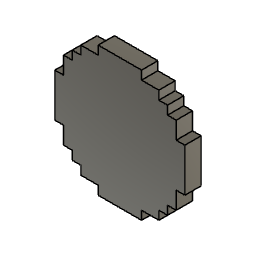
Normal Disc (Autodesk Fusion 360 design; units mm, degrees)
Autodesk Fusion 360 part; units mm, degrees
sketch "Sketch1" plane through (0, 0, 0) normal (0, 1, 0) x (1, 0, 0)
  line L0 (0, 0) -> (-8, 0)
  line L1 (0, 0) -> (0, -8)
  line L2 (0, 0) -> (8, 0)
  line L3 (8, 0) -> (8, -8)
  line L4 (8, -8) -> (0, -8)
  line L5 (0, -8) -> (0, 0)
  line L6 (8, -8) -> (8, 0)
  line L7 (8, 0) -> (16, 0)
  line L8 (16, 0) -> (16, -8)
  line L9 (16, -8) -> (8, -8)
  line L10 (16, -8) -> (16, 0)
  line L11 (16, 0) -> (24, 0)
  line L12 (24, 0) -> (24, -8)
  line L13 (24, -8) -> (16, -8)
  line L14 (24, -8) -> (24, 0)
  line L15 (24, 0) -> (32, 0)
  line L16 (32, 0) -> (32, -8)
  line L17 (32, -8) -> (24, -8)
  line L18 (32, -8) -> (32, 0)
  line L19 (32, 0) -> (40, 0)
  line L20 (40, 0) -> (40, -8)
  line L21 (40, -8) -> (32, -8)
  line L22 (40, -8) -> (40, 0)
  line L23 (40, 0) -> (48, 0)
  line L24 (48, 0) -> (48, -8)
  line L25 (48, -8) -> (40, -8)
  line L26 (48, -8) -> (48, 0)
  line L27 (48, 0) -> (56, 0)
  line L28 (56, 0) -> (56, -8)
  line L29 (56, -8) -> (48, -8)
  line L30 (56, -8) -> (56, 0)
  line L31 (56, 0) -> (64, 0)
  line L32 (64, 0) -> (64, -8)
  line L33 (64, -8) -> (56, -8)
  line L34 (64, -8) -> (64, 0)
  line L35 (64, 0) -> (72, 0)
  line L36 (72, 0) -> (72, -8)
  line L37 (72, -8) -> (64, -8)
  line L38 (72, -8) -> (72, 0)
  line L39 (72, 0) -> (80, 0)
  line L40 (80, 0) -> (80, -8)
  line L41 (80, -8) -> (72, -8)
  line L42 (80, -8) -> (80, 0)
  line L43 (80, 0) -> (88, 0)
  line L44 (88, 0) -> (88, -8)
  line L45 (88, -8) -> (80, -8)
  line L46 (88, -8) -> (88, 0)
  line L47 (88, 0) -> (96, 0)
  line L48 (96, 0) -> (96, -8)
  line L49 (96, -8) -> (88, -8)
  line L50 (96, -8) -> (96, 0)
  line L51 (96, 0) -> (104, 0)
  line L52 (104, 0) -> (104, -8)
  line L53 (104, -8) -> (96, -8)
  line L54 (104, -8) -> (104, 0)
  line L55 (104, 0) -> (112, 0)
  line L56 (112, 0) -> (112, -8)
  line L57 (112, -8) -> (104, -8)
  line L58 (112, -8) -> (112, 0)
  line L59 (112, 0) -> (120, 0)
  line L60 (120, 0) -> (120, -8)
  line L61 (120, -8) -> (112, -8)
  line L62 (32, -8) -> (32, -16)
  line L63 (72, -8) -> (72, -16)
  line L64 (8, -16) -> (8, -8)
  line L65 (32, -16) -> (32, -8)
  line L66 (64, -8) -> (64, -16)
  line L67 (80, -8) -> (80, -16)
  line L68 (32, -8) -> (40, -8)
  line L69 (8, -8) -> (16, -8)
  line L70 (56, -16) -> (56, -8)
  line L71 (80, -16) -> (80, -8)
  line L72 (64, -8) -> (72, -8)
  line L73 (96, -8) -> (96, -16)
  line L74 (48, -8) -> (56, -8)
  line L75 (88, -16) -> (88, -8)
  line L76 (48, -8) -> (48, -16)
  line L77 (0, -16) -> (0, -8)
  line L78 (104, -8) -> (104, -16)
  line L79 (88, -8) -> (88, -16)
  line L80 (24, -8) -> (32, -8)
  line L81 (16, -8) -> (24, -8)
  line L82 (8, -8) -> (8, -16)
  line L83 (0, -8) -> (8, -8)
  line L84 (88, -8) -> (96, -8)
  line L85 (24, -16) -> (24, -8)
  line L86 (48, -16) -> (48, -8)
  line L87 (56, -8) -> (64, -8)
  line L88 (16, -8) -> (16, -16)
  line L89 (24, -8) -> (24, -16)
  line L90 (80, -8) -> (88, -8)
  line L91 (96, -8) -> (104, -8)
  line L92 (40, -8) -> (40, -16)
  line L93 (72, -16) -> (72, -8)
  line L94 (104, -16) -> (104, -8)
  line L95 (64, -16) -> (64, -8)
  line L96 (40, -16) -> (40, -8)
  line L97 (104, -8) -> (112, -8)
  line L98 (96, -16) -> (96, -8)
  line L99 (72, -8) -> (80, -8)
  line L100 (56, -8) -> (56, -16)
  line L101 (16, -16) -> (16, -8)
  line L102 (0, -8) -> (0, -16)
  line L103 (40, -8) -> (48, -8)
  line L104 (104, -16) -> (96, -16)
  line L105 (112, -16) -> (104, -16)
  line L106 (96, -16) -> (88, -16)
  line L107 (64, -16) -> (56, -16)
  line L108 (120, -16) -> (112, -16)
  line L109 (24, -16) -> (16, -16)
  line L110 (88, -16) -> (80, -16)
  line L111 (56, -16) -> (48, -16)
  line L112 (72, -16) -> (64, -16)
  line L113 (80, -16) -> (72, -16)
  line L114 (40, -16) -> (32, -16)
  line L115 (32, -16) -> (24, -16)
  line L116 (8, -16) -> (0, -16)
  line L117 (48, -16) -> (40, -16)
  line L118 (16, -16) -> (8, -16)
  line L119 (120, -8) -> (120, -16)
  line L120 (112, -8) -> (120, -8)
  line L121 (112, -16) -> (112, -8)
  line L122 (32, -16) -> (32, -24)
  line L123 (72, -16) -> (72, -24)
  line L124 (8, -24) -> (8, -16)
  line L125 (32, -24) -> (32, -16)
  line L126 (64, -16) -> (64, -24)
  line L127 (80, -16) -> (80, -24)
  line L128 (32, -16) -> (40, -16)
  line L129 (8, -16) -> (16, -16)
  line L130 (56, -24) -> (56, -16)
  line L131 (80, -24) -> (80, -16)
  line L132 (64, -16) -> (72, -16)
  line L133 (96, -16) -> (96, -24)
  line L134 (48, -16) -> (56, -16)
  line L135 (88, -24) -> (88, -16)
  line L136 (48, -16) -> (48, -24)
  line L137 (0, -24) -> (0, -16)
  line L138 (104, -16) -> (104, -24)
  line L139 (88, -16) -> (88, -24)
  line L140 (24, -16) -> (32, -16)
  line L141 (16, -16) -> (24, -16)
  line L142 (8, -16) -> (8, -24)
  line L143 (0, -16) -> (8, -16)
  line L144 (88, -16) -> (96, -16)
  line L145 (24, -24) -> (24, -16)
  line L146 (48, -24) -> (48, -16)
  line L147 (56, -16) -> (64, -16)
  line L148 (16, -16) -> (16, -24)
  line L149 (24, -16) -> (24, -24)
  line L150 (80, -16) -> (88, -16)
  line L151 (96, -16) -> (104, -16)
  line L152 (40, -16) -> (40, -24)
  line L153 (72, -24) -> (72, -16)
  line L154 (104, -24) -> (104, -16)
  line L155 (64, -24) -> (64, -16)
  line L156 (40, -24) -> (40, -16)
  line L157 (104, -16) -> (112, -16)
  line L158 (96, -24) -> (96, -16)
  line L159 (72, -16) -> (80, -16)
  line L160 (56, -16) -> (56, -24)
  line L161 (16, -24) -> (16, -16)
  line L162 (0, -16) -> (0, -24)
  line L163 (40, -16) -> (48, -16)
  line L164 (104, -24) -> (96, -24)
  line L165 (112, -24) -> (104, -24)
  line L166 (96, -24) -> (88, -24)
  line L167 (64, -24) -> (56, -24)
  line L168 (120, -24) -> (112, -24)
  line L169 (24, -24) -> (16, -24)
  line L170 (88, -24) -> (80, -24)
  line L171 (56, -24) -> (48, -24)
  line L172 (72, -24) -> (64, -24)
  line L173 (80, -24) -> (72, -24)
  line L174 (40, -24) -> (32, -24)
  line L175 (32, -24) -> (24, -24)
  line L176 (8, -24) -> (0, -24)
  line L177 (48, -24) -> (40, -24)
  line L178 (16, -24) -> (8, -24)
  line L179 (120, -16) -> (120, -24)
  line L180 (112, -16) -> (120, -16)
  line L181 (112, -24) -> (112, -16)
  line L182 (32, -24) -> (32, -32)
  line L183 (72, -24) -> (72, -32)
  line L184 (8, -32) -> (8, -24)
  line L185 (32, -32) -> (32, -24)
  line L186 (64, -24) -> (64, -32)
  line L187 (80, -24) -> (80, -32)
  line L188 (32, -24) -> (40, -24)
  line L189 (8, -24) -> (16, -24)
  line L190 (56, -32) -> (56, -24)
  line L191 (80, -32) -> (80, -24)
  line L192 (64, -24) -> (72, -24)
  line L193 (96, -24) -> (96, -32)
  line L194 (48, -24) -> (56, -24)
  line L195 (88, -32) -> (88, -24)
  line L196 (48, -24) -> (48, -32)
  line L197 (0, -32) -> (0, -24)
  line L198 (104, -24) -> (104, -32)
  line L199 (88, -24) -> (88, -32)
  line L200 (24, -24) -> (32, -24)
  line L201 (16, -24) -> (24, -24)
  line L202 (8, -24) -> (8, -32)
  line L203 (0, -24) -> (8, -24)
  line L204 (88, -24) -> (96, -24)
  line L205 (24, -32) -> (24, -24)
  line L206 (48, -32) -> (48, -24)
  line L207 (56, -24) -> (64, -24)
  line L208 (16, -24) -> (16, -32)
  line L209 (24, -24) -> (24, -32)
  line L210 (80, -24) -> (88, -24)
  line L211 (96, -24) -> (104, -24)
  line L212 (40, -24) -> (40, -32)
  line L213 (72, -32) -> (72, -24)
  line L214 (104, -32) -> (104, -24)
  line L215 (64, -32) -> (64, -24)
  line L216 (40, -32) -> (40, -24)
  line L217 (104, -24) -> (112, -24)
  line L218 (96, -32) -> (96, -24)
  line L219 (72, -24) -> (80, -24)
  line L220 (56, -24) -> (56, -32)
  line L221 (16, -32) -> (16, -24)
  line L222 (0, -24) -> (0, -32)
  line L223 (40, -24) -> (48, -24)
  line L224 (104, -32) -> (96, -32)
  line L225 (112, -32) -> (104, -32)
  line L226 (96, -32) -> (88, -32)
  line L227 (64, -32) -> (56, -32)
  line L228 (120, -32) -> (112, -32)
  line L229 (24, -32) -> (16, -32)
  line L230 (88, -32) -> (80, -32)
  line L231 (56, -32) -> (48, -32)
  line L232 (72, -32) -> (64, -32)
  line L233 (80, -32) -> (72, -32)
  line L234 (40, -32) -> (32, -32)
  line L235 (32, -32) -> (24, -32)
  line L236 (8, -32) -> (0, -32)
  line L237 (48, -32) -> (40, -32)
  line L238 (16, -32) -> (8, -32)
  line L239 (120, -24) -> (120, -32)
  line L240 (112, -24) -> (120, -24)
  line L241 (112, -32) -> (112, -24)
  line L242 (32, -32) -> (32, -40)
  line L243 (72, -32) -> (72, -40)
  line L244 (8, -40) -> (8, -32)
  line L245 (32, -40) -> (32, -32)
  line L246 (64, -32) -> (64, -40)
  line L247 (80, -32) -> (80, -40)
  line L248 (32, -32) -> (40, -32)
  line L249 (8, -32) -> (16, -32)
  line L250 (56, -40) -> (56, -32)
  line L251 (80, -40) -> (80, -32)
  line L252 (64, -32) -> (72, -32)
  line L253 (96, -32) -> (96, -40)
  line L254 (48, -32) -> (56, -32)
  line L255 (88, -40) -> (88, -32)
  line L256 (48, -32) -> (48, -40)
  line L257 (0, -40) -> (0, -32)
  line L258 (104, -32) -> (104, -40)
  line L259 (88, -32) -> (88, -40)
  line L260 (24, -32) -> (32, -32)
  line L261 (16, -32) -> (24, -32)
  line L262 (8, -32) -> (8, -40)
  line L263 (0, -32) -> (8, -32)
  line L264 (88, -32) -> (96, -32)
  line L265 (24, -40) -> (24, -32)
  line L266 (48, -40) -> (48, -32)
  line L267 (56, -32) -> (64, -32)
  line L268 (16, -32) -> (16, -40)
  line L269 (24, -32) -> (24, -40)
  line L270 (80, -32) -> (88, -32)
  line L271 (96, -32) -> (104, -32)
  line L272 (40, -32) -> (40, -40)
  line L273 (72, -40) -> (72, -32)
  line L274 (104, -40) -> (104, -32)
  line L275 (64, -40) -> (64, -32)
  line L276 (40, -40) -> (40, -32)
  line L277 (104, -32) -> (112, -32)
  line L278 (96, -40) -> (96, -32)
  line L279 (72, -32) -> (80, -32)
  line L280 (56, -32) -> (56, -40)
  line L281 (16, -40) -> (16, -32)
  line L282 (0, -32) -> (0, -40)
  line L283 (40, -32) -> (48, -32)
  line L284 (104, -40) -> (96, -40)
  line L285 (112, -40) -> (104, -40)
  line L286 (96, -40) -> (88, -40)
  line L287 (64, -40) -> (56, -40)
  line L288 (120, -40) -> (112, -40)
  line L289 (24, -40) -> (16, -40)
  line L290 (88, -40) -> (80, -40)
  line L291 (56, -40) -> (48, -40)
  line L292 (72, -40) -> (64, -40)
  line L293 (80, -40) -> (72, -40)
  line L294 (40, -40) -> (32, -40)
  line L295 (32, -40) -> (24, -40)
  line L296 (8, -40) -> (0, -40)
  line L297 (48, -40) -> (40, -40)
  line L298 (16, -40) -> (8, -40)
  line L299 (120, -32) -> (120, -40)
  line L300 (112, -32) -> (120, -32)
  line L301 (112, -40) -> (112, -32)
  line L302 (32, -40) -> (32, -48)
  line L303 (72, -40) -> (72, -48)
  line L304 (8, -48) -> (8, -40)
  line L305 (32, -48) -> (32, -40)
  line L306 (64, -40) -> (64, -48)
  line L307 (80, -40) -> (80, -48)
  line L308 (32, -40) -> (40, -40)
  line L309 (8, -40) -> (16, -40)
  line L310 (56, -48) -> (56, -40)
  line L311 (80, -48) -> (80, -40)
  line L312 (64, -40) -> (72, -40)
  line L313 (96, -40) -> (96, -48)
  line L314 (48, -40) -> (56, -40)
  line L315 (88, -48) -> (88, -40)
  line L316 (48, -40) -> (48, -48)
  line L317 (0, -48) -> (0, -40)
  line L318 (104, -40) -> (104, -48)
  line L319 (88, -40) -> (88, -48)
  line L320 (24, -40) -> (32, -40)
  line L321 (16, -40) -> (24, -40)
  line L322 (8, -40) -> (8, -48)
  line L323 (0, -40) -> (8, -40)
  line L324 (88, -40) -> (96, -40)
  line L325 (24, -48) -> (24, -40)
  line L326 (48, -48) -> (48, -40)
  line L327 (56, -40) -> (64, -40)
  line L328 (16, -40) -> (16, -48)
  line L329 (24, -40) -> (24, -48)
  line L330 (80, -40) -> (88, -40)
  line L331 (96, -40) -> (104, -40)
  line L332 (40, -40) -> (40, -48)
  line L333 (72, -48) -> (72, -40)
  line L334 (104, -48) -> (104, -40)
  line L335 (64, -48) -> (64, -40)
  line L336 (40, -48) -> (40, -40)
  line L337 (104, -40) -> (112, -40)
  line L338 (96, -48) -> (96, -40)
  line L339 (72, -40) -> (80, -40)
  line L340 (56, -40) -> (56, -48)
  line L341 (16, -48) -> (16, -40)
  line L342 (0, -40) -> (0, -48)
  line L343 (40, -40) -> (48, -40)
  line L344 (104, -48) -> (96, -48)
  line L345 (112, -48) -> (104, -48)
  line L346 (96, -48) -> (88, -48)
  line L347 (64, -48) -> (56, -48)
  line L348 (120, -48) -> (112, -48)
  line L349 (24, -48) -> (16, -48)
  line L350 (88, -48) -> (80, -48)
  line L351 (56, -48) -> (48, -48)
  line L352 (72, -48) -> (64, -48)
  line L353 (80, -48) -> (72, -48)
  line L354 (40, -48) -> (32, -48)
  line L355 (32, -48) -> (24, -48)
  line L356 (8, -48) -> (0, -48)
  line L357 (48, -48) -> (40, -48)
  line L358 (16, -48) -> (8, -48)
  line L359 (120, -40) -> (120, -48)
  line L360 (112, -40) -> (120, -40)
  line L361 (112, -48) -> (112, -40)
  line L362 (32, -48) -> (32, -56)
  line L363 (72, -48) -> (72, -56)
  line L364 (8, -56) -> (8, -48)
  line L365 (32, -56) -> (32, -48)
  line L366 (64, -48) -> (64, -56)
  line L367 (80, -48) -> (80, -56)
  line L368 (32, -48) -> (40, -48)
  line L369 (8, -48) -> (16, -48)
  line L370 (56, -56) -> (56, -48)
  line L371 (80, -56) -> (80, -48)
  line L372 (64, -48) -> (72, -48)
  line L373 (96, -48) -> (96, -56)
  line L374 (48, -48) -> (56, -48)
  line L375 (88, -56) -> (88, -48)
  line L376 (48, -48) -> (48, -56)
  line L377 (0, -56) -> (0, -48)
  line L378 (104, -48) -> (104, -56)
  line L379 (88, -48) -> (88, -56)
  line L380 (24, -48) -> (32, -48)
  line L381 (16, -48) -> (24, -48)
  line L382 (8, -48) -> (8, -56)
  line L383 (0, -48) -> (8, -48)
  line L384 (88, -48) -> (96, -48)
  line L385 (24, -56) -> (24, -48)
  line L386 (48, -56) -> (48, -48)
  line L387 (56, -48) -> (64, -48)
  line L388 (16, -48) -> (16, -56)
  line L389 (24, -48) -> (24, -56)
  line L390 (80, -48) -> (88, -48)
  line L391 (96, -48) -> (104, -48)
  line L392 (40, -48) -> (40, -56)
  line L393 (72, -56) -> (72, -48)
  line L394 (104, -56) -> (104, -48)
  line L395 (64, -56) -> (64, -48)
  line L396 (40, -56) -> (40, -48)
  line L397 (104, -48) -> (112, -48)
  line L398 (96, -56) -> (96, -48)
  line L399 (72, -48) -> (80, -48)
  line L400 (56, -48) -> (56, -56)
  line L401 (16, -56) -> (16, -48)
  line L402 (0, -48) -> (0, -56)
  line L403 (40, -48) -> (48, -48)
  line L404 (104, -56) -> (96, -56)
  line L405 (112, -56) -> (104, -56)
  line L406 (96, -56) -> (88, -56)
  line L407 (64, -56) -> (56, -56)
  line L408 (120, -56) -> (112, -56)
  line L409 (24, -56) -> (16, -56)
  line L410 (88, -56) -> (80, -56)
  line L411 (56, -56) -> (48, -56)
  line L412 (72, -56) -> (64, -56)
  line L413 (80, -56) -> (72, -56)
  line L414 (40, -56) -> (32, -56)
  line L415 (32, -56) -> (24, -56)
  line L416 (8, -56) -> (0, -56)
  line L417 (48, -56) -> (40, -56)
  line L418 (16, -56) -> (8, -56)
  line L419 (120, -48) -> (120, -56)
  line L420 (112, -48) -> (120, -48)
  line L421 (112, -56) -> (112, -48)
  line L422 (32, -56) -> (32, -64)
  line L423 (72, -56) -> (72, -64)
  line L424 (8, -64) -> (8, -56)
  line L425 (32, -64) -> (32, -56)
  line L426 (64, -56) -> (64, -64)
  line L427 (80, -56) -> (80, -64)
  line L428 (32, -56) -> (40, -56)
  line L429 (8, -56) -> (16, -56)
  line L430 (56, -64) -> (56, -56)
  line L431 (80, -64) -> (80, -56)
  line L432 (64, -56) -> (72, -56)
  line L433 (96, -56) -> (96, -64)
  line L434 (48, -56) -> (56, -56)
  line L435 (88, -64) -> (88, -56)
  line L436 (48, -56) -> (48, -64)
  line L437 (0, -64) -> (0, -56)
  line L438 (104, -56) -> (104, -64)
  line L439 (88, -56) -> (88, -64)
  line L440 (24, -56) -> (32, -56)
  line L441 (16, -56) -> (24, -56)
  line L442 (8, -56) -> (8, -64)
  line L443 (0, -56) -> (8, -56)
  line L444 (88, -56) -> (96, -56)
  line L445 (24, -64) -> (24, -56)
  line L446 (48, -64) -> (48, -56)
  line L447 (56, -56) -> (64, -56)
  line L448 (16, -56) -> (16, -64)
  line L449 (24, -56) -> (24, -64)
  line L450 (80, -56) -> (88, -56)
  line L451 (96, -56) -> (104, -56)
  line L452 (40, -56) -> (40, -64)
  line L453 (72, -64) -> (72, -56)
  line L454 (104, -64) -> (104, -56)
  line L455 (64, -64) -> (64, -56)
  line L456 (40, -64) -> (40, -56)
  line L457 (104, -56) -> (112, -56)
  line L458 (96, -64) -> (96, -56)
  line L459 (72, -56) -> (80, -56)
  line L460 (56, -56) -> (56, -64)
  line L461 (16, -64) -> (16, -56)
  line L462 (0, -56) -> (0, -64)
  line L463 (40, -56) -> (48, -56)
  line L464 (104, -64) -> (96, -64)
  line L465 (112, -64) -> (104, -64)
  line L466 (96, -64) -> (88, -64)
  line L467 (64, -64) -> (56, -64)
  line L468 (120, -64) -> (112, -64)
  line L469 (24, -64) -> (16, -64)
  line L470 (88, -64) -> (80, -64)
  line L471 (56, -64) -> (48, -64)
  line L472 (72, -64) -> (64, -64)
  line L473 (80, -64) -> (72, -64)
  line L474 (40, -64) -> (32, -64)
  line L475 (32, -64) -> (24, -64)
  line L476 (8, -64) -> (0, -64)
  line L477 (48, -64) -> (40, -64)
  line L478 (16, -64) -> (8, -64)
  line L479 (120, -56) -> (120, -64)
  line L480 (112, -56) -> (120, -56)
  line L481 (112, -64) -> (112, -56)
  line L482 (32, -64) -> (32, -72)
  line L483 (72, -64) -> (72, -72)
  line L484 (8, -72) -> (8, -64)
  line L485 (32, -72) -> (32, -64)
  line L486 (64, -64) -> (64, -72)
  line L487 (80, -64) -> (80, -72)
  line L488 (32, -64) -> (40, -64)
  line L489 (8, -64) -> (16, -64)
  line L490 (56, -72) -> (56, -64)
  line L491 (80, -72) -> (80, -64)
  line L492 (64, -64) -> (72, -64)
  line L493 (96, -64) -> (96, -72)
  line L494 (48, -64) -> (56, -64)
  line L495 (88, -72) -> (88, -64)
  line L496 (48, -64) -> (48, -72)
  line L497 (0, -72) -> (0, -64)
  line L498 (104, -64) -> (104, -72)
  line L499 (88, -64) -> (88, -72)
  line L500 (24, -64) -> (32, -64)
  line L501 (16, -64) -> (24, -64)
  line L502 (8, -64) -> (8, -72)
  line L503 (0, -64) -> (8, -64)
  line L504 (88, -64) -> (96, -64)
  line L505 (24, -72) -> (24, -64)
  line L506 (48, -72) -> (48, -64)
  line L507 (56, -64) -> (64, -64)
  line L508 (16, -64) -> (16, -72)
  line L509 (24, -64) -> (24, -72)
  line L510 (80, -64) -> (88, -64)
  line L511 (96, -64) -> (104, -64)
  line L512 (40, -64) -> (40, -72)
  line L513 (72, -72) -> (72, -64)
  line L514 (104, -72) -> (104, -64)
  line L515 (64, -72) -> (64, -64)
  line L516 (40, -72) -> (40, -64)
  line L517 (104, -64) -> (112, -64)
  line L518 (96, -72) -> (96, -64)
  line L519 (72, -64) -> (80, -64)
  line L520 (56, -64) -> (56, -72)
  line L521 (16, -72) -> (16, -64)
  line L522 (0, -64) -> (0, -72)
  line L523 (40, -64) -> (48, -64)
  line L524 (104, -72) -> (96, -72)
  line L525 (112, -72) -> (104, -72)
  line L526 (96, -72) -> (88, -72)
  line L527 (64, -72) -> (56, -72)
  line L528 (120, -72) -> (112, -72)
  line L529 (24, -72) -> (16, -72)
  line L530 (88, -72) -> (80, -72)
  line L531 (56, -72) -> (48, -72)
  line L532 (72, -72) -> (64, -72)
  line L533 (80, -72) -> (72, -72)
  line L534 (40, -72) -> (32, -72)
  line L535 (32, -72) -> (24, -72)
  line L536 (8, -72) -> (0, -72)
  line L537 (48, -72) -> (40, -72)
  line L538 (16, -72) -> (8, -72)
  line L539 (120, -64) -> (120, -72)
  line L540 (112, -64) -> (120, -64)
  line L541 (112, -72) -> (112, -64)
  line L542 (32, -72) -> (32, -80)
  line L543 (72, -72) -> (72, -80)
  line L544 (8, -80) -> (8, -72)
  line L545 (32, -80) -> (32, -72)
  line L546 (64, -72) -> (64, -80)
  line L547 (80, -72) -> (80, -80)
  line L548 (32, -72) -> (40, -72)
  line L549 (8, -72) -> (16, -72)
  line L550 (56, -80) -> (56, -72)
  line L551 (80, -80) -> (80, -72)
  line L552 (64, -72) -> (72, -72)
  line L553 (96, -72) -> (96, -80)
  line L554 (48, -72) -> (56, -72)
  line L555 (88, -80) -> (88, -72)
  line L556 (48, -72) -> (48, -80)
  line L557 (0, -80) -> (0, -72)
  line L558 (104, -72) -> (104, -80)
  line L559 (88, -72) -> (88, -80)
  line L560 (24, -72) -> (32, -72)
  line L561 (16, -72) -> (24, -72)
  line L562 (8, -72) -> (8, -80)
  line L563 (0, -72) -> (8, -72)
  line L564 (88, -72) -> (96, -72)
  line L565 (24, -80) -> (24, -72)
  line L566 (48, -80) -> (48, -72)
  line L567 (56, -72) -> (64, -72)
  line L568 (16, -72) -> (16, -80)
  line L569 (24, -72) -> (24, -80)
  line L570 (80, -72) -> (88, -72)
  line L571 (96, -72) -> (104, -72)
  line L572 (40, -72) -> (40, -80)
  line L573 (72, -80) -> (72, -72)
  line L574 (104, -80) -> (104, -72)
  line L575 (64, -80) -> (64, -72)
  line L576 (40, -80) -> (40, -72)
  line L577 (104, -72) -> (112, -72)
  line L578 (96, -80) -> (96, -72)
  line L579 (72, -72) -> (80, -72)
  line L580 (56, -72) -> (56, -80)
  line L581 (16, -80) -> (16, -72)
  line L582 (0, -72) -> (0, -80)
  line L583 (40, -72) -> (48, -72)
  line L584 (104, -80) -> (96, -80)
  line L585 (112, -80) -> (104, -80)
  line L586 (96, -80) -> (88, -80)
  line L587 (64, -80) -> (56, -80)
  line L588 (120, -80) -> (112, -80)
  line L589 (24, -80) -> (16, -80)
  line L590 (88, -80) -> (80, -80)
  line L591 (56, -80) -> (48, -80)
  line L592 (72, -80) -> (64, -80)
  line L593 (80, -80) -> (72, -80)
  line L594 (40, -80) -> (32, -80)
  line L595 (32, -80) -> (24, -80)
  line L596 (8, -80) -> (0, -80)
  line L597 (48, -80) -> (40, -80)
  line L598 (16, -80) -> (8, -80)
  line L599 (120, -72) -> (120, -80)
  line L600 (112, -72) -> (120, -72)
  line L601 (112, -80) -> (112, -72)
  line L602 (32, -80) -> (32, -88)
  line L603 (72, -80) -> (72, -88)
  line L604 (8, -88) -> (8, -80)
  line L605 (32, -88) -> (32, -80)
  line L606 (64, -80) -> (64, -88)
  line L607 (80, -80) -> (80, -88)
  line L608 (32, -80) -> (40, -80)
  line L609 (8, -80) -> (16, -80)
  line L610 (56, -88) -> (56, -80)
  line L611 (80, -88) -> (80, -80)
  line L612 (64, -80) -> (72, -80)
  line L613 (96, -80) -> (96, -88)
  line L614 (48, -80) -> (56, -80)
  line L615 (88, -88) -> (88, -80)
  line L616 (48, -80) -> (48, -88)
  line L617 (0, -88) -> (0, -80)
  line L618 (104, -80) -> (104, -88)
  line L619 (88, -80) -> (88, -88)
  line L620 (24, -80) -> (32, -80)
  line L621 (16, -80) -> (24, -80)
  line L622 (8, -80) -> (8, -88)
  line L623 (0, -80) -> (8, -80)
  line L624 (88, -80) -> (96, -80)
  line L625 (24, -88) -> (24, -80)
  line L626 (48, -88) -> (48, -80)
  line L627 (56, -80) -> (64, -80)
  line L628 (16, -80) -> (16, -88)
  line L629 (24, -80) -> (24, -88)
  line L630 (80, -80) -> (88, -80)
  line L631 (96, -80) -> (104, -80)
  line L632 (40, -80) -> (40, -88)
  line L633 (72, -88) -> (72, -80)
  line L634 (104, -88) -> (104, -80)
  line L635 (64, -88) -> (64, -80)
  line L636 (40, -88) -> (40, -80)
  line L637 (104, -80) -> (112, -80)
  line L638 (96, -88) -> (96, -80)
  line L639 (72, -80) -> (80, -80)
  line L640 (56, -80) -> (56, -88)
  line L641 (16, -88) -> (16, -80)
  line L642 (0, -80) -> (0, -88)
  line L643 (40, -80) -> (48, -80)
  line L644 (104, -88) -> (96, -88)
  line L645 (112, -88) -> (104, -88)
  line L646 (96, -88) -> (88, -88)
  line L647 (64, -88) -> (56, -88)
  line L648 (120, -88) -> (112, -88)
  line L649 (24, -88) -> (16, -88)
  line L650 (88, -88) -> (80, -88)
  line L651 (56, -88) -> (48, -88)
  line L652 (72, -88) -> (64, -88)
  line L653 (80, -88) -> (72, -88)
  line L654 (40, -88) -> (32, -88)
  line L655 (32, -88) -> (24, -88)
  line L656 (8, -88) -> (0, -88)
  line L657 (48, -88) -> (40, -88)
  line L658 (16, -88) -> (8, -88)
  line L659 (120, -80) -> (120, -88)
  line L660 (112, -80) -> (120, -80)
  line L661 (112, -88) -> (112, -80)
  line L662 (32, -88) -> (32, -96)
  line L663 (72, -88) -> (72, -96)
  line L664 (8, -96) -> (8, -88)
  line L665 (32, -96) -> (32, -88)
  line L666 (64, -88) -> (64, -96)
  line L667 (80, -88) -> (80, -96)
  line L668 (32, -88) -> (40, -88)
  line L669 (8, -88) -> (16, -88)
  line L670 (56, -96) -> (56, -88)
  line L671 (80, -96) -> (80, -88)
  line L672 (64, -88) -> (72, -88)
  line L673 (96, -88) -> (96, -96)
  line L674 (48, -88) -> (56, -88)
  line L675 (88, -96) -> (88, -88)
  line L676 (48, -88) -> (48, -96)
  line L677 (0, -96) -> (0, -88)
  line L678 (104, -88) -> (104, -96)
  line L679 (88, -88) -> (88, -96)
  line L680 (24, -88) -> (32, -88)
  line L681 (16, -88) -> (24, -88)
  line L682 (8, -88) -> (8, -96)
  line L683 (0, -88) -> (8, -88)
  line L684 (88, -88) -> (96, -88)
  line L685 (24, -96) -> (24, -88)
  line L686 (48, -96) -> (48, -88)
  line L687 (56, -88) -> (64, -88)
  line L688 (16, -88) -> (16, -96)
  line L689 (24, -88) -> (24, -96)
  line L690 (80, -88) -> (88, -88)
  line L691 (96, -88) -> (104, -88)
  line L692 (40, -88) -> (40, -96)
  line L693 (72, -96) -> (72, -88)
  line L694 (104, -96) -> (104, -88)
  line L695 (64, -96) -> (64, -88)
  line L696 (40, -96) -> (40, -88)
  line L697 (104, -88) -> (112, -88)
  line L698 (96, -96) -> (96, -88)
  line L699 (72, -88) -> (80, -88)
  line L700 (56, -88) -> (56, -96)
  line L701 (16, -96) -> (16, -88)
  line L702 (0, -88) -> (0, -96)
  line L703 (40, -88) -> (48, -88)
  line L704 (104, -96) -> (96, -96)
  line L705 (112, -96) -> (104, -96)
  line L706 (96, -96) -> (88, -96)
  line L707 (64, -96) -> (56, -96)
  line L708 (120, -96) -> (112, -96)
  line L709 (24, -96) -> (16, -96)
  line L710 (88, -96) -> (80, -96)
  line L711 (56, -96) -> (48, -96)
  line L712 (72, -96) -> (64, -96)
  line L713 (80, -96) -> (72, -96)
  line L714 (40, -96) -> (32, -96)
  line L715 (32, -96) -> (24, -96)
  line L716 (8, -96) -> (0, -96)
  line L717 (48, -96) -> (40, -96)
  line L718 (16, -96) -> (8, -96)
  line L719 (120, -88) -> (120, -96)
  line L720 (112, -88) -> (120, -88)
  line L721 (112, -96) -> (112, -88)
  line L722 (32, -96) -> (32, -104)
  line L723 (72, -96) -> (72, -104)
  line L724 (8, -104) -> (8, -96)
  line L725 (32, -104) -> (32, -96)
  line L726 (64, -96) -> (64, -104)
  line L727 (80, -96) -> (80, -104)
  line L728 (32, -96) -> (40, -96)
  line L729 (8, -96) -> (16, -96)
  line L730 (56, -104) -> (56, -96)
  line L731 (80, -104) -> (80, -96)
  line L732 (64, -96) -> (72, -96)
  line L733 (96, -96) -> (96, -104)
  line L734 (48, -96) -> (56, -96)
  line L735 (88, -104) -> (88, -96)
  line L736 (48, -96) -> (48, -104)
  line L737 (0, -104) -> (0, -96)
  line L738 (104, -96) -> (104, -104)
  line L739 (88, -96) -> (88, -104)
  line L740 (24, -96) -> (32, -96)
  line L741 (16, -96) -> (24, -96)
  line L742 (8, -96) -> (8, -104)
  line L743 (0, -96) -> (8, -96)
  line L744 (88, -96) -> (96, -96)
  line L745 (24, -104) -> (24, -96)
  line L746 (48, -104) -> (48, -96)
  line L747 (56, -96) -> (64, -96)
  line L748 (16, -96) -> (16, -104)
  line L749 (24, -96) -> (24, -104)
  line L750 (80, -96) -> (88, -96)
  line L751 (96, -96) -> (104, -96)
  line L752 (40, -96) -> (40, -104)
  line L753 (72, -104) -> (72, -96)
  line L754 (104, -104) -> (104, -96)
  line L755 (64, -104) -> (64, -96)
  line L756 (40, -104) -> (40, -96)
  line L757 (104, -96) -> (112, -96)
  line L758 (96, -104) -> (96, -96)
  line L759 (72, -96) -> (80, -96)
  line L760 (56, -96) -> (56, -104)
  line L761 (16, -104) -> (16, -96)
  line L762 (0, -96) -> (0, -104)
  line L763 (40, -96) -> (48, -96)
  line L764 (104, -104) -> (96, -104)
  line L765 (112, -104) -> (104, -104)
  line L766 (96, -104) -> (88, -104)
  line L767 (64, -104) -> (56, -104)
  line L768 (120, -104) -> (112, -104)
  line L769 (24, -104) -> (16, -104)
  line L770 (88, -104) -> (80, -104)
  line L771 (56, -104) -> (48, -104)
  line L772 (72, -104) -> (64, -104)
  line L773 (80, -104) -> (72, -104)
  line L774 (40, -104) -> (32, -104)
  line L775 (32, -104) -> (24, -104)
  line L776 (8, -104) -> (0, -104)
  line L777 (48, -104) -> (40, -104)
  line L778 (16, -104) -> (8, -104)
  line L779 (120, -96) -> (120, -104)
  line L780 (112, -96) -> (120, -96)
  line L781 (112, -104) -> (112, -96)
  line L782 (32, -104) -> (32, -112)
  line L783 (72, -104) -> (72, -112)
  line L784 (8, -112) -> (8, -104)
  line L785 (32, -112) -> (32, -104)
  line L786 (64, -104) -> (64, -112)
  line L787 (80, -104) -> (80, -112)
  line L788 (32, -104) -> (40, -104)
  line L789 (8, -104) -> (16, -104)
  line L790 (56, -112) -> (56, -104)
  line L791 (80, -112) -> (80, -104)
  line L792 (64, -104) -> (72, -104)
  line L793 (96, -104) -> (96, -112)
  line L794 (48, -104) -> (56, -104)
  line L795 (88, -112) -> (88, -104)
  line L796 (48, -104) -> (48, -112)
  line L797 (0, -112) -> (0, -104)
  line L798 (104, -104) -> (104, -112)
  line L799 (88, -104) -> (88, -112)
  line L800 (24, -104) -> (32, -104)
  line L801 (16, -104) -> (24, -104)
  line L802 (8, -104) -> (8, -112)
  line L803 (0, -104) -> (8, -104)
  line L804 (88, -104) -> (96, -104)
  line L805 (24, -112) -> (24, -104)
  line L806 (48, -112) -> (48, -104)
  line L807 (56, -104) -> (64, -104)
  line L808 (16, -104) -> (16, -112)
  line L809 (24, -104) -> (24, -112)
  line L810 (80, -104) -> (88, -104)
  line L811 (96, -104) -> (104, -104)
  line L812 (40, -104) -> (40, -112)
  line L813 (72, -112) -> (72, -104)
  line L814 (104, -112) -> (104, -104)
  line L815 (64, -112) -> (64, -104)
  line L816 (40, -112) -> (40, -104)
  line L817 (104, -104) -> (112, -104)
  line L818 (96, -112) -> (96, -104)
  line L819 (72, -104) -> (80, -104)
  line L820 (56, -104) -> (56, -112)
  line L821 (16, -112) -> (16, -104)
  line L822 (0, -104) -> (0, -112)
  line L823 (40, -104) -> (48, -104)
  line L824 (104, -112) -> (96, -112)
  line L825 (112, -112) -> (104, -112)
  line L826 (96, -112) -> (88, -112)
  line L827 (64, -112) -> (56, -112)
  line L828 (120, -112) -> (112, -112)
  line L829 (24, -112) -> (16, -112)
  line L830 (88, -112) -> (80, -112)
  line L831 (56, -112) -> (48, -112)
  line L832 (72, -112) -> (64, -112)
  line L833 (80, -112) -> (72, -112)
  line L834 (40, -112) -> (32, -112)
  line L835 (32, -112) -> (24, -112)
  line L836 (8, -112) -> (0, -112)
  line L837 (48, -112) -> (40, -112)
  line L838 (16, -112) -> (8, -112)
  line L839 (120, -104) -> (120, -112)
  line L840 (112, -104) -> (120, -104)
  line L841 (112, -112) -> (112, -104)
  line L842 (32, -112) -> (32, -120)
  line L843 (72, -112) -> (72, -120)
  line L844 (8, -120) -> (8, -112)
  line L845 (32, -120) -> (32, -112)
  line L846 (64, -112) -> (64, -120)
  line L847 (80, -112) -> (80, -120)
  line L848 (32, -112) -> (40, -112)
  line L849 (8, -112) -> (16, -112)
  line L850 (56, -120) -> (56, -112)
  line L851 (80, -120) -> (80, -112)
  line L852 (64, -112) -> (72, -112)
  line L853 (96, -112) -> (96, -120)
  line L854 (48, -112) -> (56, -112)
  line L855 (88, -120) -> (88, -112)
  line L856 (48, -112) -> (48, -120)
  line L857 (0, -120) -> (0, -112)
  line L858 (104, -112) -> (104, -120)
  line L859 (88, -112) -> (88, -120)
  line L860 (24, -112) -> (32, -112)
  line L861 (16, -112) -> (24, -112)
  line L862 (8, -112) -> (8, -120)
  line L863 (0, -112) -> (8, -112)
  line L864 (88, -112) -> (96, -112)
  line L865 (24, -120) -> (24, -112)
  line L866 (48, -120) -> (48, -112)
  line L867 (56, -112) -> (64, -112)
  line L868 (16, -112) -> (16, -120)
  line L869 (24, -112) -> (24, -120)
  line L870 (80, -112) -> (88, -112)
  line L871 (96, -112) -> (104, -112)
  line L872 (40, -112) -> (40, -120)
  line L873 (72, -120) -> (72, -112)
  line L874 (104, -120) -> (104, -112)
  line L875 (64, -120) -> (64, -112)
  line L876 (40, -120) -> (40, -112)
  line L877 (104, -112) -> (112, -112)
  line L878 (96, -120) -> (96, -112)
  line L879 (72, -112) -> (80, -112)
  line L880 (56, -112) -> (56, -120)
  line L881 (16, -120) -> (16, -112)
  line L882 (0, -112) -> (0, -120)
  line L883 (40, -112) -> (48, -112)
  line L884 (104, -120) -> (96, -120)
  line L885 (112, -120) -> (104, -120)
  line L886 (96, -120) -> (88, -120)
  line L887 (64, -120) -> (56, -120)
  line L888 (120, -120) -> (112, -120)
  line L889 (24, -120) -> (16, -120)
  line L890 (88, -120) -> (80, -120)
  line L891 (56, -120) -> (48, -120)
  line L892 (72, -120) -> (64, -120)
  line L893 (80, -120) -> (72, -120)
  line L894 (40, -120) -> (32, -120)
  line L895 (32, -120) -> (24, -120)
  line L896 (8, -120) -> (0, -120)
  line L897 (48, -120) -> (40, -120)
  line L898 (16, -120) -> (8, -120)
  line L899 (120, -112) -> (120, -120)
  line L900 (112, -112) -> (120, -112)
  line L901 (112, -120) -> (112, -112)
  point P0 (0, -8)
  point P1 (0, -8)
  point P2 (0, -16)
  point P3 (0, -16)
  point P4 (0, -24)
  point P5 (0, -24)
  point P6 (0, -32)
  point P7 (0, -32)
  point P8 (0, -40)
  point P9 (0, -40)
  point P10 (0, -48)
  point P11 (0, -48)
  point P12 (0, -56)
  point P13 (0, -56)
  point P14 (0, -64)
  point P15 (0, -64)
  point P16 (0, -72)
  point P17 (0, -72)
  point P18 (0, -80)
  point P19 (0, -80)
  point P20 (0, -88)
  point P21 (0, -88)
  point P22 (0, -96)
  point P23 (0, -96)
  point P24 (0, -104)
  point P25 (0, -104)
  point P26 (0, -112)
  point P27 (0, -112)
  dimension "d1" = 8
  dimension "d4" = 112
  dimension "d5" = 0
  dimension "d8" = 0
  dimension "d9" = -8
  constraint coincident L0.start L1.start
  constraint horizontal L0
  constraint perpendicular L0 L1
  constraint equal L0 L1
  constraint horizontal L2
  constraint vertical L3
  constraint horizontal L4
  constraint vertical L5
  constraint equal L0 L2
  constraint equal L0 L5
  measures "d1" distance of L0.start L0.end
extrude "Extrude2" add sketch "Sketch1" along normal blind 15 contours L17 L62 L65 L80 L85 L89 L115 L140 | L109 L141 L145 L148 L149 L161 L169 L201 | L178 L184 L189 L202 L208 L221 L238 L249 | L21 L62 L65 L68 L92 L96 L114 L128 | L115 L122 L125 L140 L145 L149 L175 L200 | L169 L201 L205 L208 L209 L221 L229 L261 | L238 L244 L249 L262 L268 L281 L298 L309 | L296 L304 L317 L322 L323 L342 L356 L383 | L20 L22 L23 L24 L25 L26 L103 | L25 L76 L86 L92 L96 L103 L117 L163 | L114 L122 L125 L128 L152 L156 L174 L188 | L175 L182 L185 L200 L205 L209 L235 L260 | L229 L261 L265 L268 L269 L281 L289 L321 | L298 L304 L309 L322 L328 L341 L358 L369 | L356 L364 L377 L382 L383 L402 L416 L443 | L24 L26 L27 L28 L29 L30 L74 | L29 L70 L74 L76 L86 L100 L111 L134 | L117 L136 L146 L152 L156 L163 L177 L223 | L174 L182 L185 L188 L212 L216 L234 L248 | L235 L242 L245 L260 L265 L269 L295 L320 | L289 L321 L325 L328 L329 L341 L349 L381 | L358 L364 L369 L382 L388 L401 L418 L429 | L416 L424 L437 L442 L443 L462 L476 L503 | L28 L30 L31 L32 L33 L34 L87 | L33 L66 L70 L87 L95 L100 L107 L147 | L111 L130 L134 L136 L146 L160 L171 L194 | L177 L196 L206 L212 L216 L223 L237 L283 | L234 L242 L245 L248 L272 L276 L294 L308 | L295 L302 L305 L320 L325 L329 L355 L380 | L349 L381 L385 L388 L389 L401 L409 L441 | L418 L424 L429 L442 L448 L461 L478 L489 | L476 L484 L497 L502 L503 L522 L536 L563 | L32 L34 L35 L36 L37 L38 L72 | L37 L63 L66 L72 L93 L95 L112 L132 | L107 L126 L130 L147 L155 L160 L167 L207 | L171 L190 L194 L196 L206 L220 L231 L254 | L237 L256 L266 L272 L276 L283 L297 L343 | L294 L302 L305 L308 L332 L336 L354 L368 | L355 L362 L365 L380 L385 L389 L415 L440 | L409 L441 L445 L448 L449 L461 L469 L501 | L478 L484 L489 L502 L508 L521 L538 L549 | L536 L544 L557 L562 L563 L582 L596 L623 | L36 L38 L39 L40 L41 L42 L99 | L41 L63 L67 L71 L93 L99 L113 L159 | L112 L123 L126 L132 L153 L155 L172 L192 | L167 L186 L190 L207 L215 L220 L227 L267 | L231 L250 L254 L256 L266 L280 L291 L314 | L297 L316 L326 L332 L336 L343 L357 L403 | L354 L362 L365 L368 L392 L396 L414 L428 | L415 L422 L425 L440 L445 L449 L475 L500 | L469 L501 L505 L508 L509 L521 L529 L561 | L538 L544 L549 L562 L568 L581 L598 L609 | L45 L67 L71 L75 L79 L90 L110 L150 | L113 L123 L127 L131 L153 L159 L173 L219 | L172 L183 L186 L192 L213 L215 L232 L252 | L227 L246 L250 L267 L275 L280 L287 L327 | L291 L310 L314 L316 L326 L340 L351 L374 | L357 L376 L386 L392 L396 L403 L417 L463 | L414 L422 L425 L428 L452 L456 L474 L488 | L475 L482 L485 L500 L505 L509 L535 L560 | L529 L561 L565 L568 L569 L581 L589 L621 | L598 L604 L609 L622 L628 L641 L658 L669 | L49 L73 L75 L79 L84 L98 L106 L144 | L110 L127 L131 L135 L139 L150 L170 L210 | L173 L183 L187 L191 L213 L219 L233 L279 | L232 L243 L246 L252 L273 L275 L292 L312 | L287 L306 L310 L327 L335 L340 L347 L387 | L351 L370 L374 L376 L386 L400 L411 L434 | L417 L436 L446 L452 L456 L463 L477 L523 | L474 L482 L485 L488 L512 L516 L534 L548 | L535 L542 L545 L560 L565 L569 L595 L620 | L589 L621 L625 L628 L629 L641 L649 L681 | L658 L664 L669 L682 L688 L701 L718 L729 | L106 L133 L135 L139 L144 L158 L166 L204 | L170 L187 L191 L195 L199 L210 L230 L270 | L233 L243 L247 L251 L273 L279 L293 L339 | L292 L303 L306 L312 L333 L335 L352 L372 | L347 L366 L370 L387 L395 L400 L407 L447 | L411 L430 L434 L436 L446 L460 L471 L494 | L477 L496 L506 L512 L516 L523 L537 L583 | L534 L542 L545 L548 L572 L576 L594 L608 | L595 L602 L605 L620 L625 L629 L655 L680 | L649 L681 L685 L688 L689 L701 L709 L741 | L104 L133 L138 L151 L154 L158 L164 L211 | L166 L193 L195 L199 L204 L218 L226 L264 | L230 L247 L251 L255 L259 L270 L290 L330 | L293 L303 L307 L311 L333 L339 L353 L399 | L352 L363 L366 L372 L393 L395 L412 L432 | L407 L426 L430 L447 L455 L460 L467 L507 | L471 L490 L494 L496 L506 L520 L531 L554 | L537 L556 L566 L572 L576 L583 L597 L643 | L594 L602 L605 L608 L632 L636 L654 L668 | L655 L662 L665 L680 L685 L689 L715 L740 | L709 L741 L745 L748 L749 L761 L769 L801 | L164 L193 L198 L211 L214 L218 L224 L271 | L226 L253 L255 L259 L264 L278 L286 L324 | L290 L307 L311 L315 L319 L330 L350 L390 | L353 L363 L367 L371 L393 L399 L413 L459 | L412 L423 L426 L432 L453 L455 L472 L492 | L467 L486 L490 L507 L515 L520 L527 L567 | L531 L550 L554 L556 L566 L580 L591 L614 | L597 L616 L626 L632 L636 L643 L657 L703 | L654 L662 L665 L668 L692 L696 L714 L728 | L715 L722 L725 L740 L745 L749 L775 L800 | L165 L198 L214 L217 L225 L241 L277 | L224 L253 L258 L271 L274 L278 L284 L331 | L286 L313 L315 L319 L324 L338 L346 L384 | L350 L367 L371 L375 L379 L390 L410 L450 | L413 L423 L427 L431 L453 L459 L473 L519 | L472 L483 L486 L492 L513 L515 L532 L552 | L527 L546 L550 L567 L575 L580 L587 L627 | L591 L610 L614 L616 L626 L640 L651 L674 | L657 L676 L686 L692 L696 L703 L717 L763 | L714 L722 L725 L728 L752 L756 L774 L788 | L775 L782 L785 L800 L805 L809 L835 L860 | L225 L258 L274 L277 L285 L301 L337 | L284 L313 L318 L331 L334 L338 L344 L391 | L346 L373 L375 L379 L384 L398 L406 L444 | L410 L427 L431 L435 L439 L450 L470 L510 | L473 L483 L487 L491 L513 L519 L533 L579 | L532 L543 L546 L552 L573 L575 L592 L612 | L587 L606 L610 L627 L635 L640 L647 L687 | L651 L670 L674 L676 L686 L700 L711 L734 | L717 L736 L746 L752 L756 L763 L777 L823 | L774 L782 L785 L788 L812 L816 L834 L848 | L285 L318 L334 L337 L345 L361 L397 | L344 L373 L378 L391 L394 L398 L404 L451 | L406 L433 L435 L439 L444 L458 L466 L504 | L470 L487 L491 L495 L499 L510 L530 L570 | L533 L543 L547 L551 L573 L579 L593 L639 | L592 L603 L606 L612 L633 L635 L652 L672 | L647 L666 L670 L687 L695 L700 L707 L747 | L711 L730 L734 L736 L746 L760 L771 L794 | L777 L796 L806 L812 L816 L823 L837 L883 | L288 L348 L359 L360 L361 L420 | L345 L378 L394 L397 L405 L421 L457 | L404 L433 L438 L451 L454 L458 L464 L511 | L466 L493 L495 L499 L504 L518 L526 L564 | L530 L547 L551 L555 L559 L570 L590 L630 | L593 L603 L607 L611 L633 L639 L653 L699 | L652 L663 L666 L672 L693 L695 L712 L732 | L707 L726 L730 L747 L755 L760 L767 L807 | L771 L790 L794 L796 L806 L820 L831 L854 | L837 L856 L866 L872 L876 L883 L897 | L348 L408 L419 L420 L421 L480 | L405 L438 L454 L457 L465 L481 L517 | L464 L493 L498 L511 L514 L518 L524 L571 | L526 L553 L555 L559 L564 L578 L586 L624 | L590 L607 L611 L615 L619 L630 L650 L690 | L653 L663 L667 L671 L693 L699 L713 L759 | L712 L723 L726 L732 L753 L755 L772 L792 | L767 L786 L790 L807 L815 L820 L827 L867 | L831 L850 L854 L856 L866 L880 L891 | L408 L468 L479 L480 L481 L540 | L465 L498 L514 L517 L525 L541 L577 | L524 L553 L558 L571 L574 L578 L584 L631 | L586 L613 L615 L619 L624 L638 L646 L684 | L650 L667 L671 L675 L679 L690 L710 L750 | L713 L723 L727 L731 L753 L759 L773 L819 | L772 L783 L786 L792 L813 L815 L832 L852 | L827 L846 L850 L867 L875 L880 L887 | L468 L528 L539 L540 L541 L600 | L525 L558 L574 L577 L585 L601 L637 | L584 L613 L618 L631 L634 L638 L644 L691 | L646 L673 L675 L679 L684 L698 L706 L744 | L710 L727 L731 L735 L739 L750 L770 L810 | L773 L783 L787 L791 L813 L819 L833 L879 | L832 L843 L846 L852 L873 L875 L892 | L528 L588 L599 L600 L601 L660 | L585 L618 L634 L637 L645 L661 L697 | L644 L673 L678 L691 L694 L698 L704 L751 | L706 L733 L735 L739 L744 L758 L766 L804 | L770 L787 L791 L795 L799 L810 L830 L870 | L833 L843 L847 L851 L873 L879 L893 | L645 L678 L694 L697 L705 L721 L757 | L704 L733 L738 L751 L754 L758 L764 L811 | L766 L793 L795 L799 L804 L818 L826 L864
